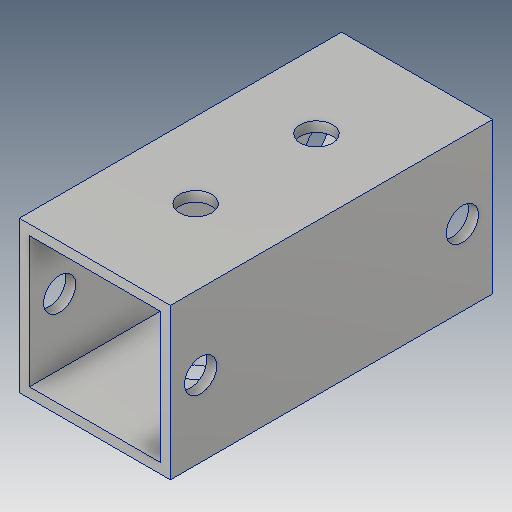
# Autodesk Inventor part: 支え角柱(サーボ用)
Saved by Autodesk Inventor 2019.4 (Build 234330000, 330)
## iProperties
Created: 2019-06-16
Part Number: 支え角柱(サーボ用)
Material: アルミニウム 6061
Document SubType Name: Modeling
Designer: 長谷川翔一
Density: 2.7 g/cm^3
Appearance: アルミニウム - フラット
Mass: 4.75154 g
Surface Area: 36.7187 cm^2
Volume: 1.75983 cm^3
Author: 長谷川翔一
Autodesk Inventor part; units mm, degrees
ref_plane "YZ Plane" through (0, 0, 0) normal (1, 0, 0) x (0, 1, 0)
ref_plane "XZ Plane" through (0, 0, 0) normal (0, 1, 0) x (-1, 0, 0)
ref_plane "XY Plane" through (0, 0, 0) normal (0, 0, 1) x (1, 0, 0)
sketch "スケッチ1" plane through (0, 0, 0) normal (0, 0, 1) x (1, 0, 0)
  line L0 (7.5, -7.5) -> (-7.5, -7.5)
  line L1 (-7.5, -7.5) -> (-7.5, 7.5)
  line L2 (-7.5, 7.5) -> (7.5, 7.5)
  line L3 (7.5, 7.5) -> (7.5, -7.5)
  line L4 (7.5, -7.5) -> (-7.5, 7.5) construction
  line L5 (-7.5, -7.5) -> (7.5, 7.5) construction
  line L6 (-7.5, 0) -> (7.5, 0) construction
  line L7 (6.5, 6.5) -> (-6.5, 6.5)
  line L8 (-6.5, 6.5) -> (-6.5, -6.5)
  line L9 (-6.5, -6.5) -> (6.5, -6.5)
  line L10 (6.5, -6.5) -> (6.5, 6.5)
  point P0 (0, 0)
  dimension "d0" = 15
  dimension "d1" = 15
  dimension "d2" = 1
  constraints: 22 end point, 4 midpoint, 4 parallel, 2 perpendicular, 1 horizontal, 3 other
  measures "d0" distance of L1.end L2.end
  measures "d1" distance of L0.end L1.end
  measures "d2" distance between parallel lines of L2 L7
extrude "押し出し1" add sketch "スケッチ1" along normal blind 32
sketch "スケッチ2" plane through (7.5, -7.5, 0) normal (1, 0, 0) x (0, 0, -1)
  line L0 (0, 15) -> (0, 0) projected
  line L1 (0, 15) -> (-32, 15) projected
  line L2 (-32, 0) -> (-32, 15) projected
  line L3 (0, 0) -> (-32, 0) projected
  line L4 (-32, 7.5) -> (0, 7.5) construction
  line L5 (-16, 7.5) -> (-16, 15) construction
  circle A0 centre (-29, 7.5) radius 3 construction
  circle A1 centre (-29, 7.5) radius 1.6
  circle A2 centre (-3, 7.5) radius 3 construction
  circle A3 centre (-3, 7.5) radius 1.6
  dimension "d5" = 6
  dimension "d6" = 3.2
  constraints: 4 centre point, 4 end point, 3 midpoint, 2 coincident, 2 symmetric about line, 1 horizontal, 1 point on line, 1 tangent, 2 other
  measures "d5" diameter of A0
  measures "d6" diameter of A1
extrude "押し出し2" cut sketch "スケッチ2" against normal through all contours A1 | A3
sketch "スケッチ3" plane through (-7.5, 7.5, 0) normal (0, 1, 0) x (1, 0, 0)
  line L0 (0, 0) -> (15, 0) projected
  line L1 (0, 0) -> (0, -32) projected
  line L2 (15, -32) -> (0, -32) projected
  line L3 (15, 0) -> (15, -32) projected
  line L4 (7.5, 0) -> (7.5, -32) construction
  line L5 (15, -16) -> (0, -16) construction
  circle A0 centre (7.5, -10) radius 1.6
  circle A1 centre (7.5, -22) radius 1.6
  dimension "d9" = 3.2
  dimension "d10" = 6
  constraints: 4 end point, 3 midpoint, 2 centre point, 1 point on line, 1 symmetric about line, 1 other
  measures "d9" diameter of A0
  measures "d10" distance from line of A0.centre L5
extrude "押し出し3" cut sketch "スケッチ3" against normal through all contours A0 | A1
